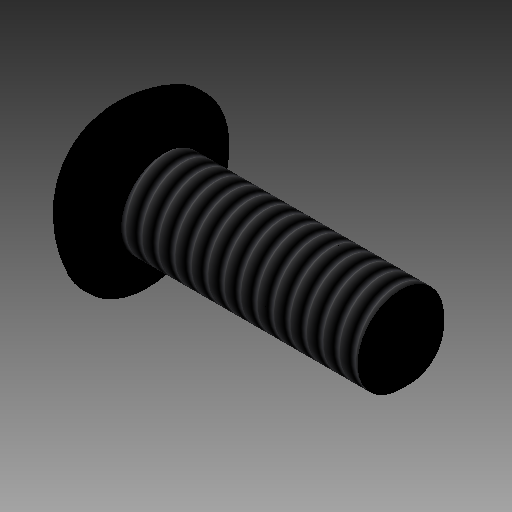
# Autodesk Inventor part: 3024
Saved by Autodesk Inventor 2019 (Build 230136000, 136)
## iProperties
Category: PARTsolutions
Company: 8020
Created: 2018-10-13
Part Number: 3024
Material: Generic
Catalog Web Link: www.cadenas.de
Description: 3005, 3024, 3032, 3042, 3050, 3051, 3054, 3059, 3061, 3063, 3065, 3104, 3111, 3114, 3117, 3118-Button Head Socket Cap Screws
Vendor: 8020
Document SubType Name: Modeling
Designer: psadmin
Manufacturer: 8020
Mass: 0.240488 g
Surface Area: 3.02581 cm^2
Volume: 0.240488 cm^3
Density: 1 g/cm^3
Appearance: PSOLRGB-0-0-0
PSOL_IDENT_0: {$CADENAS_DATA\23d-libs\8020\inch\fastening_options\3005.prj},238 {VTYP=3D},{NB=3024},{LINA=3024},{N
PSOL_IDENT_1: N=3005, 3024, 3032, 3042, 3050, 3051, 3054, 3059, 3061, 3063, 3065, 3104, 3111, 3114, 3117, 3118},{D
PSOL_IDENT_2: ATE=02.07.2018 05:48:01},{GEOMDATE=03.08.2012 12:04:00},{VERSION=},{LINEID=10},{WBVAR=L},{WBNUMERIC=
PSOL_IDENT_3: L}  {NB=3024},{LINA=3024},{KT=DUMMY},{PN=3024},{FIN=Black Zinc},{THRD=8-32},{THRD1=0.1640},{L=0.5000
PSOL_IDENT_4: 0000},{L1=[0.375,0.5,0.875]},{TT=UNC},{A=0.313},{A1=0.3125},{H=0.087},{H1=0.011},{J=0.094},{J1=0.093
PSOL_IDENT_5: 75},{T=0.0781},{R=0.175},{W=.003}
NN: 3005, 3024, 3032, 3042, 3050, 3051, 3054, 3059, 3061, 3063, 3065, 3104, 3111, 3114, 3117, 3118
NT: Button Head Socket Cap Screws
NB: 3024
NBSYN: $PN.
LINA: 3024
PN: 3024
FIN: Black Zinc
THRD: 8-32
L: 0
A: 0.313
H: 0.087
J: 0.094
W: .003
SUPPLIER: 8020
ARTICLENO: 3024
BOMINFO: 3024
CREATOR: CADENAS GmbH
d5: 0.000 in
d6: 0.000 in
Title: 3024
Author: Cadenas PARTsolutions
Comments: Button Head Socket Cap Screws
Autodesk Inventor part; units mm, degrees
sketch "Sketch_1" plane through (0, 0, 0) normal (0, 0, 1) x (1, 0, 0)
  line L0 (12.7, 0) -> (-2.2098, 0)
  line L1 (-2.2098, 0) -> (-2.2098, 2.0828)
  arc A0 (-0.2794, 3.9688) -> (-2.2098, 2.0828) centre (1.7151, -0.0037) ccw
  line L2 (-0.2794, 3.9688) -> (0, 3.9688)
  line L3 (0, 3.9688) -> (0, 2.0828)
  line L4 (0, 2.0828) -> (12.2276, 2.0828)
  line L5 (12.2276, 2.0828) -> (12.7, 1.6104)
  line L6 (12.7, 1.6104) -> (12.7, 0)
  line L7 (12.7, 0) -> (-2.2098, 0)
  constraints: 16 end point, 2 point on circle, 1 centre point
revolve "Revolution1" add sketch "Sketch_1" angle 360 about axis through (12.7, 0, 0) along (1, 0, 0)
thread "Thread1" size "8-32 UNC" class "2A" standard "ANSI Unified Screw Threads" length 11.4093
sketch "Sketch_3" plane through (-2.2098, 0, 0) normal (1, 0, 0) x (0, 0, -1)
  line L0 (-1.3748, 0) -> (-0.6874, -1.1906)
  line L1 (-0.6874, -1.1906) -> (0.6874, -1.1906)
  line L2 (0.6874, -1.1906) -> (1.3748, 0)
  line L3 (1.3748, 0) -> (0.6874, 1.1906)
  line L4 (0.6874, 1.1906) -> (-0.6874, 1.1906)
  line L5 (-0.6874, 1.1906) -> (-1.3748, 0)
  constraints: 12 end point
extrude "Extrusion1" cut sketch "Sketch_3" along normal mid plane 3.9675
ref_plane "screw_XY" through (0, 0, 0) normal (1, 0, 0) x (0, 0, -1)
ref_plane "screw_YZ" through (0, 0, 0) normal (0, 0, -1) x (0, 1, 0)
ref_plane "screw_ZX" through (0, 0, 0) normal (0, 1, 0) x (1, 0, 0)
ref_plane "to_nut_XY" through (12.7, 0, 0) normal (1, 0, 0) x (0, 0, -1)
ref_plane "to_nut_YZ" through (12.7, 0, 0) normal (0, 0, -1) x (0, 1, 0)
ref_plane "to_nut_ZX" through (12.7, 0, 0) normal (0, 1, 0) x (1, 0, 0)
body "Solid1"
